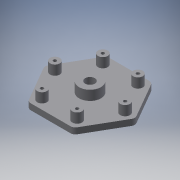
# Autodesk Inventor part: rotor 2
Saved by Autodesk Inventor 2017 (Build 210142000, 142)
## iProperties
Created: 2018-01-19
Part Number: rotor 2
Material: Generic
Document SubType Name: Modeling
Designer: RLanting
Density: 1 g/cm^3
Appearance: Default
Author: RLanting
Autodesk Inventor part; units mm, degrees
ref_plane "YZ Plane" through (0, 0, 0) normal (1, 0, 0) x (0, 1, 0)
ref_plane "XZ Plane" through (0, 0, 0) normal (0, 1, 0) x (-1, 0, 0)
ref_plane "XY Plane" through (0, 0, 0) normal (0, 0, 1) x (1, 0, 0)
sketch "Sketch1" plane through (0, 0, 0) normal (0, 0, 1) x (1, 0, 0)
  line L0 (-14.5, 25.1147) -> (14.5, 25.1147) construction
  line L1 (14.5, 25.1147) -> (29, 0) construction
  line L2 (29, 0) -> (14.5, -25.1147) construction
  line L3 (14.5, -25.1147) -> (-14.5, -25.1147) construction
  line L4 (-14.5, -25.1147) -> (-29, 0) construction
  line L5 (-29, 0) -> (-14.5, 25.1147) construction
  line L6 (-18.7639, 32.5) -> (18.7639, 32.5)
  line L7 (18.7639, 32.5) -> (37.5278, 0)
  line L8 (37.5278, 0) -> (18.7639, -32.5)
  line L9 (18.7639, -32.5) -> (-18.7639, -32.5)
  line L10 (-18.7639, -32.5) -> (-37.5278, 0)
  line L11 (-37.5278, 0) -> (-18.7639, 32.5)
  circle A0 centre (-14.5, 25.1147) radius 11 construction
  circle A1 centre (14.5, 25.1147) radius 11 construction
  circle A2 centre (29, 0) radius 11 construction
  circle A3 centre (14.5, -25.1147) radius 11 construction
  circle A4 centre (-14.5, -25.1147) radius 11 construction
  circle A5 centre (-29, 0) radius 11 construction
  circle A6 centre (-14.5, 25.1147) radius 4
  circle A7 centre (14.5, 25.1147) radius 4
  circle A8 centre (29, 0) radius 4
  circle A9 centre (14.5, -25.1147) radius 4
  circle A10 centre (-14.5, -25.1147) radius 4
  circle A11 centre (-29, 0) radius 4
  circle A12 centre (0, 0) radius 4
  circle A13 centre (0, 0) radius 40 construction
  circle A14 centre (0, 0) radius 37.5278 construction
  dimension "d17" = 75.0555
  dimension "d0" = 22
  dimension "d1" = 50.2295
  dimension "d2" = 8
  dimension "d3" = 65
  dimension "d4" = 8
  dimension "d13" = 80
  constraints: 24 end point, 17 coincident, 14 centre point, 10 equal radius, 2 horizontal, 1 tangent, 29 other
  measures "d0" diameter of A0
  measures "d1" distance between parallel lines of L3 L0
  measures "d2" diameter of A6
  measures "d3" distance between parallel lines of L9 L6
  measures "d4" diameter of A12
  measures "d13" diameter of A13
extrude "Extrusion1" add sketch "Sketch1" along normal blind 5
fillet "Fillet1" radius 4 6 edges at (37.5278, 0, 2.5) (18.7639, -32.5, 2.5) (-18.7639, -32.5, 2.5) (-37.5278, 0, 2.5) (-18.7639, 32.5, 2.5) (18.7639, 32.5, 2.5)
sketch "Sketch2" plane through (0, 0, 5) normal (0, 0, 1) x (1, 0, 0)
  arc A0 (19.9186, 30.5) -> (16.4545, 32.5) centre (16.4545, 28.5) ccw projected
  line L0 (16.4545, 32.5) -> (-16.4545, 32.5) projected
  arc A1 (-16.4545, 32.5) -> (-19.9186, 30.5) centre (-16.4545, 28.5) ccw projected
  line L1 (-19.9186, 30.5) -> (-36.3731, 2) projected
  arc A2 (-36.3731, 2) -> (-36.3731, -2) centre (-32.909, 0) ccw projected
  line L2 (-36.3731, -2) -> (-19.9186, -30.5) projected
  arc A3 (-19.9186, -30.5) -> (-16.4545, -32.5) centre (-16.4545, -28.5) ccw projected
  line L3 (-16.4545, -32.5) -> (16.4545, -32.5) projected
  arc A4 (16.4545, -32.5) -> (19.9186, -30.5) centre (16.4545, -28.5) ccw projected
  line L4 (19.9186, -30.5) -> (36.3731, -2) projected
  arc A5 (36.3731, -2) -> (36.3731, 2) centre (32.909, 0) ccw projected
  line L5 (36.3731, 2) -> (19.9186, 30.5) projected
  circle A6 centre (0, 0) radius 4 projected
  circle A7 centre (-29, 0) radius 4 projected
  circle A8 centre (-14.5, -25.1147) radius 4 projected
  circle A9 centre (14.5, -25.1147) radius 4 projected
  circle A10 centre (29, 0) radius 4 projected
  circle A11 centre (14.5, 25.1147) radius 4 projected
  circle A12 centre (-14.5, 25.1147) radius 4 projected
  circle A13 centre (0, 0) radius 4 projected
  circle A14 centre (0, 0) radius 9
  dimension "d8" = 5
  constraints: 1 centre point, 1 coincident
  measures "d8" radial gap between concentric circles of A6 A14
extrude "Extrusion2" add sketch "Sketch2" along normal blind 8 contours A7 | A8 | A9 | A10 | A11 | A12 | A14
sketch "Sketch3" plane through (0, 0, 0) normal (0, 0, -1) x (-1, 0, 0)
  circle A0 centre (0, 0) radius 4 projected
  circle A1 centre (29, 0) radius 4 projected
  circle A2 centre (14.5, -25.1147) radius 4 projected
  circle A3 centre (-14.5, -25.1147) radius 4 projected
  circle A4 centre (-29, 0) radius 4 projected
  circle A5 centre (-14.5, 25.1147) radius 4 projected
  circle A6 centre (14.5, 25.1147) radius 4 projected
  arc A7 (-16.4545, 32.5) -> (-19.9186, 30.5) centre (-16.4545, 28.5) ccw projected
  line L0 (-19.9186, 30.5) -> (-36.3731, 2) projected
  arc A8 (-36.3731, 2) -> (-36.3731, -2) centre (-32.909, 0) ccw projected
  line L1 (-36.3731, -2) -> (-19.9186, -30.5) projected
  arc A9 (-19.9186, -30.5) -> (-16.4545, -32.5) centre (-16.4545, -28.5) ccw projected
  line L2 (-16.4545, -32.5) -> (16.4545, -32.5) projected
  arc A10 (16.4545, -32.5) -> (19.9186, -30.5) centre (16.4545, -28.5) ccw projected
  line L3 (19.9186, -30.5) -> (36.3731, -2) projected
  arc A11 (36.3731, -2) -> (36.3731, 2) centre (32.909, 0) ccw projected
  line L4 (36.3731, 2) -> (19.9186, 30.5) projected
  arc A12 (19.9186, 30.5) -> (16.4545, 32.5) centre (16.4545, 28.5) ccw projected
  line L5 (16.4545, 32.5) -> (-16.4545, 32.5) projected
extrude "Extrusion3" add sketch "Sketch3" against normal up to next contours A1 | A2 | A3 | A4 | A5 | A6
sketch "Sketch4" plane through (0, 0, 0) normal (0, 0, -1) x (-1, 0, 0)
  circle A0 centre (-14.5, 25.1147) radius 4 construction
  circle A1 centre (14.5, 25.1147) radius 4 construction
  circle A2 centre (29, 0) radius 4 construction
  circle A3 centre (14.5, -25.1147) radius 4 construction
  circle A4 centre (-14.5, -25.1147) radius 4 construction
  circle A5 centre (-29, 0) radius 4 construction
  circle A6 centre (-14.5, 25.1147) radius 1.35
  circle A7 centre (14.5, 25.1147) radius 1.35
  circle A8 centre (29, 0) radius 1.35
  circle A9 centre (14.5, -25.1147) radius 1.35
  circle A10 centre (-14.5, -25.1147) radius 1.35
  circle A11 centre (-29, 0) radius 1.35
  point P0 (0, 0)
  dimension "d14" = 2.7
  constraints: 6 centre point, 6 coincident, 5 equal radius
  measures "d14" diameter of A6
extrude "Extrusion4" cut sketch "Sketch4" against normal through all
body "Solid1"
